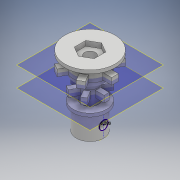
# Autodesk Inventor part: wheelSpindle
Saved by Autodesk Inventor 2018 (Build 220112000, 112)
## iProperties
Created: 2017-10-22
Part Number: wheelSpindle
Material: Generic
Document SubType Name: Modeling
Designer: Prakash
Density: 1 g/cm^3
Appearance: Default
Author: Prakash
Autodesk Inventor part; units mm, degrees
ref_plane "XZ Plane" through (0, 0, 0) normal (0, 1, 0) x (-1, 0, 0)
ref_plane "XY Plane" through (0, 0, 0) normal (0, 0, 1) x (1, 0, 0)
sketch "Sketch1" plane through (0, 0, 0) normal (0, 0, 1) x (1, 0, 0)
  circle A0 centre (0, 0) radius 5
  circle A1 centre (0, 0) radius 10
  circle A2 centre (0, 0) radius 3.175
  circle A3 centre (0, 0) radius 8.175
  dimension "d18" = 6.35
  dimension "d19" = 16.35
  dimension "d40" = 10
  dimension "d41" = 5
  constraints: 4 centre point, 4 coincident
  measures "d18" diameter of A2
  measures "d19" diameter of A3
  measures "d40" diameter of A0
  measures "d41" radial gap between concentric circles of A1 A0
extrude "Extrusion1" add sketch "Sketch1" along normal blind 14 contours A0 | A2
extrude "Extrusion2" add sketch "Sketch1" along normal blind 2 contours A1 | A3
extrude "Extrusion5" cut sketch "Sketch1" along normal up to surface (14 mm away) contours A2
extrude "Extrusion6" add sketch "Sketch1" against normal blind 14 contours A0 | A3
ref_plane "Work Plane2" through (8.175, 0, 0) normal (1, 0, 0) x (0, 1, 0)
sketch "Sketch10" plane through (8.175, 0, 0) normal (1, 0, 0) x (0, 1, 0)
  line L0 (0, 0) -> (0, -14) construction
  line L1 (3.175, -14) -> (-3.175, -14) construction
  circle A0 centre (0, -7) radius 2.6543
  circle A1 centre (0, -7) radius 2.5273
  dimension "d67" = 5.3086
  dimension "d68" = 5.0546
  constraints: 2 centre point, 2 end point, 2 midpoint, 1 coincident
  measures "d67" diameter of A0
  measures "d68" diameter of A1
extrude "Extrusion10" cut sketch "Sketch10" against normal blind 3.81 contours A1
loft "Loft1" cut profiles "Sketch10" section 2 edges at (4.365, -2.5273, -7) contours A0 | A1
hole "Hole2" at (8.175, 0, -7) direction (-1, 0, 0) diameter 3.797 end up to face face through (0, 0, 0) facing (0, 0, 1) round with radius 3.175 far side yes clearance for "Flat Head Machine Screw (82)" size "#6" standard "Ansi Unified Screw Threads"
sketch "Sketch11" plane through (0, 0, 14) normal (0, 0, 1) x (1, 0, 0)
  circle A0 centre (0, 0) radius 3.175 projected
  circle A1 centre (0, 0) radius 3.175
  circle A2 centre (0, 0) radius 10
  dimension "d82" = 20
  constraints: 2 centre point, 2 coincident, 1 concentric
  measures "d82" diameter of A2
extrude "Extrusion11" add sketch "Sketch11" along normal blind 12
sketch "Sketch12" plane through (0, 0, 26) normal (0, 0, 1) x (1, 0, 0)
  circle A0 centre (0, 0) radius 10 projected
  circle A1 centre (0, 0) radius 15
  circle A2 centre (0, 0) radius 3.175 projected
  circle A3 centre (0, 0) radius 3.175
  dimension "d85" = 5
  constraints: 2 centre point, 1 coincident
  measures "d85" radial gap between concentric circles of A0 A1
extrude "Extrusion12" add sketch "Sketch12" along normal blind 2 contours A0 | A1
ref_plane "Work Plane3" through (0, 0, 20) normal (0, 0, -1) x (-1, 0, 0)
ref_plane "Work Plane4" through (0, 0, 8) normal (0, 0, -1) x (-1, 0, 0)
sketch "Sketch13" plane through (0, 0, 20) normal (0, 0, -1) x (-1, 0, 0)
  circle A0 centre (0, 0) radius 10 projected
  circle A1 centre (0, 0) radius 10
  line L0 (-10, 0) -> (-15, 0)
  line L1 (-15, 0) -> (-15, 2)
  line L2 (-15, 0) -> (-15, -2)
  line L3 (0, 0) -> (-10, 0)
  line L4 (-15, -2) -> (-9.798, -2)
  line L5 (-15, 2) -> (-9.798, 2)
  circle A2 centre (0, 0) radius 15 projected
  circle A3 centre (0, 0) radius 10 projected
  point P0 (-12.5, 0)
  dimension "d89" = 2
  dimension "d90" = 2
  dimension "d96" = 5
  constraints: 12 end point, 3 horizontal, 3 point on circle, 2 coincident, 1 centre point, 1 concentric, 1 midpoint, 1 parallel, 1 perpendicular, 1 vertical
  measures "d89" distance of L0.end L1.end
  measures "d90" distance of L0.end L2.end
  measures "d96" distance of L0.start L0.end
extrude "Extrusion13" add sketch "Sketch13" along normal mid plane 4 contours A0 L0 A2 L5 | L4 A2 L0 A0 | A2 L1 L5 | L4 L2 A2
sketch "Sketch14" plane through (0, 0, 8) normal (0, 0, -1) x (-1, 0, 0)
  circle A0 centre (0, 0) radius 5 projected
  line L0 (-5, 0) -> (-10, 0)
  line L1 (0, 0) -> (-5, 0)
  line L2 (-10, 0) -> (-10, 1.5)
  line L3 (-10, 0) -> (-10, -1.5)
  line L4 (-10, -1.5) -> (-4.7697, -1.5)
  line L5 (-10, 1.5) -> (-4.7697, 1.5)
  dimension "d93" = 1.5
  dimension "d94" = 1.5
  dimension "d95" = 5
  constraints: 12 end point, 3 point on circle, 2 horizontal, 2 vertical, 1 parallel, 1 perpendicular
  measures "d93" distance of L0.end L2.end
  measures "d94" distance of L0.end L3.end
  measures "d95" distance of L0.start L0.end
extrude "Extrusion14" add sketch "Sketch14" along normal mid plane 4 contours A0 L0 L2 L5 | L4 L3 L0 A0
fillet "Fillet2" radius 3.75 2 edges at (-10, 0, 14) (-5, 0, 14)
pattern_circular "Circular Pattern1" count 6 over 360 about axis through (0, 0, 17.75) along (0, 0, -1) of "Extrusion13"
pattern_circular "Circular Pattern2" count 6 over 360 about axis through (0, 0, 17.75) along (0, 0, -1) of "Extrusion14"
sketch "Sketch15" plane through (0, 0, 28) normal (0, 0, 1) x (1, 0, 0)
  line L0 (6, 3.4641) -> (6, -3.4641)
  line L1 (6, -3.4641) -> (0, -6.9282)
  line L2 (0, -6.9282) -> (-6, -3.4641)
  line L3 (-6, -3.4641) -> (-6, 3.4641)
  line L4 (-6, 3.4641) -> (0, 6.9282)
  line L5 (0, 6.9282) -> (6, 3.4641)
  point P0 (0, 0)
  point P1 (0, 0)
  dimension "d106" = 12
  constraints: 12 end point, 1 coincident, 1 vertical, 13 other
  measures "d106" distance between parallel lines of L2 L5
extrude "Extrusion15" cut sketch "Sketch15" against normal blind 3
sketch "Sketch16" plane through (0, 0, -14) normal (0, 0, -1) x (-1, 0, 0)
  circle A0 centre (0, 0) radius 4.7625
  circle A1 centre (0, 0) radius 3.175 projected
  circle A2 centre (0, 0) radius 3.175
  dimension "d109" = 9.525
  constraints: 2 centre point, 2 coincident
  measures "d109" diameter of A0
extrude "Extrusion16" cut sketch "Sketch16" against normal blind 1.5
equation "\"d94\" = d93"
body "Solid1"
